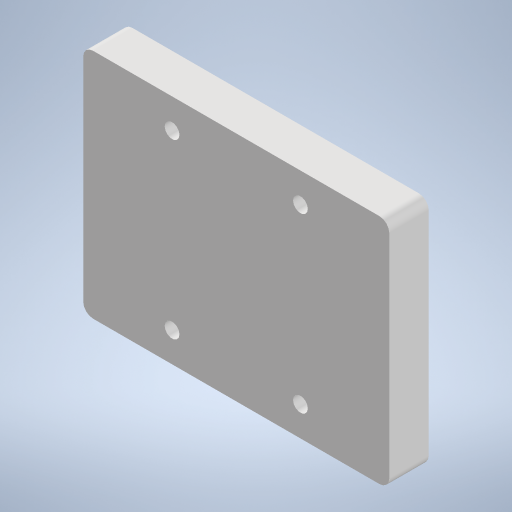
# Autodesk Inventor part: uchwyt_2
Saved by Autodesk Inventor 2023 (Build 270158000, 158)
## iProperties
Created: 2022-11-07
Part Number: uchwyt_2
Material: Generic
Document SubType Name: Modeling
Designer: Kamil
Density: 1 g/cm^3
Appearance: Default
Author: Kamil
Autodesk Inventor part; units mm, degrees
ref_plane "YZ Plane" through (0, 0, 0) normal (1, 0, 0) x (0, 1, 0)
ref_plane "XZ Plane" through (0, 0, 0) normal (0, 1, 0) x (-1, 0, 0)
ref_plane "XY Plane" through (0, 0, 0) normal (0, 0, 1) x (1, 0, 0)
sketch "Sketch9" plane through (0, 0, 0) normal (0, 0, 1) x (1, 0, 0)
  line L0 (44, 0) -> (44, -29)
  line L1 (0, -29) -> (0, 0)
  line L2 (44, 0) -> (38, 0)
  line L3 (0, -29) -> (6, -29)
  circle A0 centre (9, -32) radius 1.5
  circle A1 centre (35, -32) radius 1.5
  circle A2 centre (35, 3) radius 1.5
  circle A3 centre (9, 3) radius 1.5
  line L4 (0, 0) -> (0, 10)
  line L5 (0, 10) -> (-10, 10)
  line L6 (44, -29) -> (54, -29)
  line L7 (54, -29) -> (54, -39)
  line L8 (-10, 10) -> (54, 10)
  line L9 (54, 10) -> (54, -39)
  line L10 (54, -39) -> (-10, -39)
  line L11 (-10, -39) -> (-10, 10)
  line L12 (-10, 10) -> (-10, 13)
  line L13 (-10, 13) -> (-13, 13)
  line L14 (54, -39) -> (54, -42)
  line L15 (54, -42) -> (57, -42)
  line L16 (57, -42) -> (-13, -42)
  line L17 (-13, -42) -> (-13, 13)
  line L18 (-13, 13) -> (57, 13)
  line L19 (57, 13) -> (57, -42)
  circle A4 centre (9, 3) radius 3
  circle A5 centre (35, 3) radius 3
  circle A6 centre (35, -32) radius 3
  circle A7 centre (9, -32) radius 3
  dimension "d22" = 3
  dimension "d23" = 3
  dimension "d24" = 3
  dimension "d25" = 3
  dimension "d26" = 6
  dimension "d27" = 6
  dimension "d29" = 6
  dimension "d30" = 6
  constraints: 40 end point, 8 centre point, 6 perpendicular, 5 parallel, 4 coincident, 3 horizontal, 3 vertical
  measures "d22" distance of L5.end L12.end
  measures "d23" distance of L12.end L13.end
  measures "d24" distance of L7.end L14.end
  measures "d25" distance of L14.end L15.end
  measures "d26" diameter of A4
  measures "d27" diameter of A5
  measures "d29" diameter of A6
  measures "d30" diameter of A7
extrude "Extrusion1" add sketch "Sketch9" along normal blind 3 contours L8 L9 L7 L10 L11 L5 | L5 L12 L18 L19 L15 L14 L7 L9 L8 | L11 L10 L14 L16 L17 L13 L12
sketch "Sketch10" plane through (0, 0, 3) normal (0, 0, 1) x (1, 0, 0)
  line L0 (57, -42) -> (57, 13) projected
  line L1 (57, 11) -> (57, 10)
  line L2 (57, 13) -> (-13, 13) projected
  line L3 (55, 13) -> (54, 13)
  line L4 (54, 13) -> (54, 10)
  line L5 (57, 10) -> (57, 9)
  line L6 (54, 13) -> (53, 13)
  line L7 (53, 13) -> (53, 9)
  line L8 (-13, 13) -> (-13, -42) projected
  line L9 (-13, -40) -> (-13, -38)
  arc A0 (-13, -40) -> (-11, -42) centre (-11, -40) ccw projected
  line L10 (-11, -42) -> (-9, -42)
  line L11 (-13, -38) -> (-9, -38)
  line L12 (-9, -38) -> (-9, -42)
  line L13 (-9, -42) -> (-13, -42)
  line L14 (-13, -42) -> (-13, -38)
  line L15 (-9, -38) -> (53, -38)
  line L16 (53, -38) -> (53, 9)
  line L17 (53, 9) -> (-9, 9)
  line L18 (-9, 9) -> (-9, -38)
  line L19 (-13, -38) -> (-9, -38)
  line L20 (-9, -38) -> (-9, -42)
  line L21 (-9, -42) -> (-13, -42)
  line L22 (-13, -42) -> (-13, -38)
  line L23 (-9, 9) -> (53, 9)
  line L24 (53, 9) -> (53, -38)
  line L25 (53, -38) -> (-9, -38)
  line L26 (-9, -38) -> (-9, 9)
  line L27 (-13.4447, 13.4817) -> (58.1663, 13.4817)
  line L28 (58.1663, 13.4817) -> (58.1663, -42.7185)
  line L29 (58.1663, -42.7185) -> (-13.4447, -42.7185)
  line L30 (-13.4447, -42.7185) -> (-13.4447, 13.4817)
  line L31 (-9, 9) -> (53, 9)
  line L32 (53, 9) -> (53, -38)
  line L33 (53, -38) -> (-9, -38)
  line L34 (-9, -38) -> (-9, 9)
  line L35 (-14.6617, 14.1825) -> (60.6079, 14.1825)
  line L36 (60.6079, 14.1825) -> (60.6079, -44.8629)
  line L37 (60.6079, -44.8629) -> (-14.6617, -44.8629)
  line L38 (-14.6617, -44.8629) -> (-14.6617, 14.1825)
  point P0 (0, 0)
  point P1 (57, -40)
  point P2 (-11, 13)
  point P3 (-13, 11)
  point P4 (-13, -40)
  point P5 (-13, -40)
  dimension "d36" = 1
  dimension "d37" = 1
  dimension "d38" = 1
  dimension "d39" = 1
  dimension "d40" = 2
  dimension "d41" = 2
  constraints: 72 end point, 14 parallel, 9 perpendicular, 8 horizontal, 5 point on line, 1 tangent
  measures "d36" distance of L1.start L1.end
  measures "d37" distance of L3.start L3.end
  measures "d38" distance of L1.end L5.end
  measures "d39" distance of L3.end L6.end
  measures "d40" distance of L9.start L9.end
  measures "d41" distance of L10.start L10.end
extrude "Extrusion4" cut sketch "Sketch10" against normal blind 6 contours L7 L17 L18 L11 L8 L2 | L11 L12 L10 A0 L8 | L27 L28 L29 L30
sketch "Sketch27" plane through (0, 0, 3) normal (0, 0, 1) x (1, 0, 0)
  point P0 (0, 0)
sketch "Sketch28" plane through (0, 0, 3) normal (0, 0, 1) x (1, 0, 0)
  line L0 (-9, 9) -> (53, 9)
  line L1 (53, 9) -> (53, -38)
  line L2 (53, -38) -> (-9, -38)
  line L3 (-9, -38) -> (-9, 9)
  point P0 (0, 0)
  constraints: 8 end point, 2 parallel, 1 horizontal, 1 perpendicular
extrude "Extrusion7" add sketch "Sketch28" along normal blind 3
extrude "Extrusion8" cut sketch "Sketch9" against normal blind 6 contours A0 | A1 | A2 | A3
extrude "Extrusion9" cut sketch "Sketch9" along normal blind 82.9 contours A0 | A1 | A2 | A3
sketch "Sketch29" plane through (0, 0, 0) normal (0, 0, -1) x (-1, 0, 0)
  line L0 (17.5138, -45.6881) -> (10.4067, -45.6881)
  line L1 (10.4067, -45.6881) -> (10.4067, -38.0734)
  line L2 (10.4067, -38.0734) -> (17.5138, -38.0734)
  line L3 (17.5138, -38.0734) -> (17.5138, -45.6881)
  point P0 (0, 0)
  constraints: 8 end point, 2 parallel, 1 horizontal, 1 perpendicular
extrude "Extrusion10" cut sketch "Sketch29" against normal blind 25.05
sketch "Sketch30" plane through (0, 0, 0) normal (0, 0, -1) x (-1, 0, 0)
  line L0 (-53, -38) -> (9, -38) projected
  line L1 (9, -38) -> (-53, -38)
  line L2 (-53, -38) -> (-53, 9.1187)
  line L3 (-53, 9.1187) -> (9, 9.1187)
  line L4 (9, 9.1187) -> (9, -38)
  point P0 (0, 0)
  constraints: 8 end point, 2 parallel, 1 horizontal, 1 perpendicular
sketch "Sketch31" plane through (0, 0, 0) normal (0, 0, -1) x (-1, 0, 0)
  circle A0 centre (-9, -32) radius 3 projected
  circle A1 centre (-9, -32) radius 4
  circle A2 centre (-35, -32) radius 1.5 projected
  circle A3 centre (-9, 3) radius 3 projected
  circle A4 centre (-9, 3) radius 4
  circle A5 centre (-35, 3) radius 3 projected
  circle A6 centre (-35, 3) radius 4
  point P0 (0, 0)
  constraints: 3 centre point, 3 coincident
extrude "Extrusion11" add sketch "Sketch30" along normal blind 2
extrude "Extrusion12" cut sketch "Sketch31" along normal blind 2 contours A0 | A3 | A5
sketch "Sketch32" plane through (0, 0, -2) normal (0, 0, -1) x (-1, 0, 0)
  point P0 (0, 0)
extrude "Extrusion14" cut sketch "Sketch31" along normal blind 8 contours A2
extrude "Extrusion15" cut sketch "Sketch9" against normal blind 4 contours A1 | A6
sketch "Sketch34" plane through (0, 0, -2) normal (0, 0, -1) x (-1, 0, 0)
  point P0 (0, 0)
sketch "Sketch35" plane through (0, 0, -2) normal (0, 0, -1) x (-1, 0, 0)
  line L0 (-53, -38) -> (-53, 9) projected
  line L1 (9, -38) -> (-53, -38)
  line L2 (-53, -38) -> (-53, 9)
  line L3 (-53, 9) -> (9, 9)
  line L4 (9, 9) -> (9, -38)
  line L5 (9, 9.1187) -> (-53, 9.1187) projected
  line L6 (9, 9) -> (-53, 9)
  line L7 (-53, 9) -> (-53, 9.1187)
  line L8 (-53, 9.1187) -> (9, 9.1187)
  line L9 (9, 9.1187) -> (9, 9)
  point P0 (0, 0)
  constraints: 16 end point, 4 parallel, 2 horizontal, 2 perpendicular
extrude "Extrusion16" cut sketch "Sketch35" against normal blind 4 contours L7 L5 L9 L3
fillet "Fillet4" radius 2 4 edges at (-9, -38, 2) (53, -38, 2) (53, 9, 2) (-9, 9, 2)
body "Solid1"
